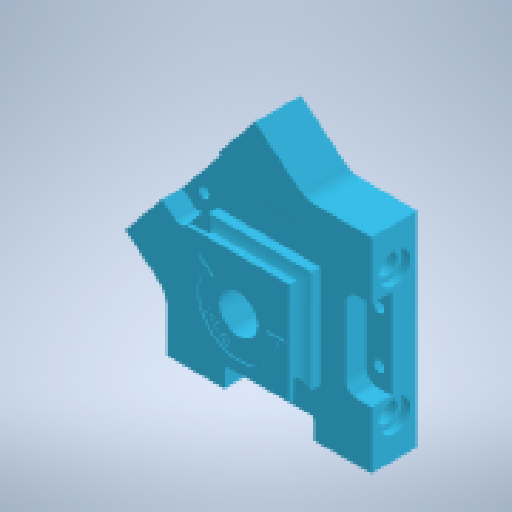
# Autodesk Inventor part: Rail-Angle140.66
Saved by Autodesk Inventor 2023.1 (Build 271208000, 208)
## iProperties
Created: 2023-06-07
Part Number: Rail-Angle140.66
Material: ABS Plastic
Document SubType Name: Modeling
Designer: hello
Density: 1.06 g/cm^3
Appearance: Turquoise
Author: hello
Autodesk Inventor part; units mm, degrees
ref_plane "YZ Plane" through (0, 0, 0) normal (1, 0, 0) x (0, 1, 0)
ref_plane "XZ Plane" through (0, 0, 0) normal (0, 1, 0) x (-1, 0, 0)
ref_plane "XY Plane" through (0, 0, 0) normal (0, 0, 1) x (1, 0, 0)
sketch "Sketch1" plane through (0, 0, 0) normal (0, 0, 1) x (1, 0, 0)
  line L0 (-40, 40) -> (40, 40)
  line L1 (40, 40) -> (40, -40)
  line L2 (40, -40) -> (-40, -40)
  line L3 (-40, -40) -> (-40, 40)
  line L4 (-40, 40) -> (40, -40) construction
  line L5 (40, 40) -> (-40, -40) construction
  line L6 (-56.2928, -5.5791) -> (-5.5791, 56.2928)
  line L7 (40, 0) -> (-40, 0) construction
  line L8 (0, 0) -> (-30.9359, 25.3568) construction
  line L9 (-56.2928, -5.5791) -> (-40, -18.9335)
  line L10 (-5.5791, 56.2928) -> (14.2984, 40)
  dimension "d0" = 80
  dimension "d1" = 80
  dimension "d2" = 80
  dimension "d3" = 140.66
  dimension "d4" = 40
  constraints: 22 end point, 5 midpoint, 4 perpendicular, 2 horizontal, 2 parallel, 2 point on line
  measures "d0" distance of L1.end L2.end
  measures "d1" distance of L0.end L1.end
  measures "d2" distance of L6.start L6.end
  measures "d3" angle of L8 L7
  measures "d4" distance of L8.start L8.end
extrude "Extrusion1" add sketch "Sketch1" along normal blind 18 contours L0 L1 L2 L3 L6 | L0 L6 L10 | L3 L9 L6
sketch "Sketch2" plane through (40, -40, 0) normal (1, 0, 0) x (0, 0, -1)
  line L0 (0, 0) -> (0, 80) projected
  line L1 (0, 80) -> (-18, 80) projected
  line L2 (-18, 0) -> (-18, 80) projected
  line L3 (0, 0) -> (-18, 0) projected
  line L4 (-9, 15) -> (-9, 65)
  point P0 (0, 40)
  point P1 (-9, 40)
  point P2 (0, 40)
  point P3 (-9, 0)
  dimension "d7" = 50
  constraints: 3 midpoint, 2 coincident, 2 end point, 1 horizontal alignment, 1 vertical, 1 vertical alignment
  measures "d7" distance of L4.start L4.end
hole "Hole1" at (40, -25, 9) at (40, 25, 9) direction (-1, 0, 0) diameter 8.05 depth 15 counterbore diameter 12 counterbore depth 3
sketch "Sketch3" plane through (-40, -40, 0) normal (0, -1, 0) x (1, 0, 0)
  line L0 (0, 0) -> (80, 0) projected
  line L1 (80, 0) -> (80, 18) projected
  line L2 (0, 18) -> (80, 18) projected
  line L3 (0, 0) -> (0, 18) projected
  line L4 (15, 9) -> (65, 9)
  point P0 (40, 0)
  point P1 (40, 9)
  point P2 (0, 9)
  point P3 (40, 0)
  dimension "d15" = 50
  constraints: 3 midpoint, 2 coincident, 2 end point, 1 horizontal, 1 horizontal alignment, 1 vertical alignment
  measures "d15" distance of L4.start L4.end
hole "Hole2" at (-25, -40, 9) at (25, -40, 9) direction (0, 1, 0) diameter 8.05 depth 15 counterbore diameter 12 counterbore depth 3
sketch "Sketch4" plane through (0, 0, 18) normal (0, 0, 1) x (1, 0, 0)
  line L0 (40, -40) -> (40, 40) projected
  line L1 (34, -17.5) -> (40, -17.5)
  line L2 (40, -17.5) -> (40, 17.5)
  line L3 (40, 17.5) -> (34, 17.5)
  line L4 (30, 13.5) -> (30, -13.5)
  arc A0 (30, -13.5) -> (34, -17.5) centre (34, -13.5) ccw
  arc A1 (34, 17.5) -> (30, 13.5) centre (34, 13.5) ccw
  point P0 (0, 0)
  point P1 (30, -17.5)
  point P2 (30, 17.5)
  point P3 (40, 0)
  dimension "d23" = 35
  dimension "d24" = 10
  dimension "d25" = 4
  constraints: 8 end point, 4 point on circle, 4 point on line, 4 tangent, 2 centre point, 2 midpoint, 2 parallel, 1 equal radius, 1 horizontal, 1 perpendicular
  measures "d23" distance of point (30, 17.5) point (30, -17.5)
  measures "d24" distance of point (30, -17.5) L1.end
  measures "d25" radius of A0
extrude "Extrusion2" cut sketch "Sketch4" against normal blind 8
sketch "Sketch5" plane through (0, 0, 10) normal (0, 0, 1) x (1, 0, 0)
  line L0 (35, -10) -> (35, 10)
  line L1 (40, 17.5) -> (40, -17.5) projected
  point P0 (0, 0)
  point P1 (35, 0)
  point P2 (40, 0)
  dimension "d28" = 20
  dimension "d29" = 5
  constraints: 2 coincident, 2 end point, 2 midpoint, 1 horizontal alignment, 1 vertical
  measures "d28" distance of L0.start L0.end
  measures "d29" distance between parallel lines of L1 L0
hole "Hole3" at (35, -10, 10) at (35, 10, 10) direction (0, 0, -1) diameter 4 depth 5
pattern_circular "Circular Pattern1" count 2 over 90 about axis through (0, 0, -10) along (0, 0, -1) of "Extrusion2", "Hole3"
sketch "Sketch6" plane through (0, 0, 18) normal (0, 0, 1) x (1, 0, 0)
  line L0 (-20, 20) -> (20, 20)
  line L1 (20, 20) -> (20, -20)
  line L2 (20, -20) -> (-20, -20)
  line L3 (-20, -20) -> (-20, 20)
  line L4 (-20, 20) -> (20, -20) construction
  line L5 (20, 20) -> (-20, -20) construction
  point P0 (0, 0)
  dimension "d40" = 40
  dimension "d41" = 40
  constraints: 12 end point, 2 midpoint, 2 parallel, 1 horizontal, 1 perpendicular
  measures "d40" distance of L1.end L2.end
  measures "d41" distance of L0.end L1.end
extrude "Extrusion3" add sketch "Sketch6" along normal blind 12
sketch "Sketch7" plane through (-56.2928, -5.5791, 0) normal (-0.7733978, 0.633921, 0) x (0, 0, 1)
  line L0 (0, 80) -> (0, 0) projected
  line L1 (0, 0) -> (18, 0) projected
  line L2 (18, 80) -> (18, 0) projected
  line L3 (0, 80) -> (18, 80) projected
  line L4 (9, 65) -> (9, 15)
  point P0 (0, 40)
  point P1 (9, 40)
  point P2 (0, 40)
  point P3 (9, 80)
  dimension "d44" = 50
  constraints: 3 midpoint, 2 coincident, 2 end point, 1 horizontal alignment, 1 vertical, 1 vertical alignment
  measures "d44" distance of L4.start L4.end
hole "Hole4" at (-15.0879, 44.6918, 9) at (-46.7839, 6.0219, 9) direction (0.7733978, -0.633921, 0) diameter 8.05 depth 15 counterbore diameter 12 counterbore depth 3
sketch "Sketch9" plane through (0, 0, 18) normal (0, 0, 1) x (1, 0, 0)
  line L0 (-14.644, 29.4585) -> (-31.7599, 8.5768)
  line L1 (-37.3891, 8.0189) -> (-42.0295, 11.8224)
  line L2 (-42.0295, 11.8224) -> (-19.8423, 38.8913)
  line L3 (-19.8423, 38.8913) -> (-15.2019, 35.0878)
  line L4 (-12.1083, 32.5521) -> (-42.0295, 11.8224) construction
  line L5 (-34.2956, 5.4832) -> (-19.8423, 38.8913) construction
  line L6 (-5.5791, 56.2928) -> (-56.2928, -5.5791) projected
  arc A0 (-14.644, 29.4585) -> (-15.2019, 35.0878) centre (-17.7376, 31.9942) ccw
  arc A1 (-37.3891, 8.0189) -> (-31.7599, 8.5768) centre (-34.8535, 11.1124) ccw
  point P0 (0, 0)
  point P1 (-27.0689, 22.1872)
  point P2 (-30.9359, 25.3568)
  dimension "d52" = 10
  dimension "d53" = 35
  dimension "d56" = 4
  constraints: 12 end point, 4 midpoint, 4 point on circle, 4 point on line, 4 tangent, 2 centre point, 2 parallel, 1 collinear, 1 equal radius, 1 perpendicular
  measures "d52" distance of L5.start L1.end
  measures "d53" distance of L4.start L5.start
  measures "d56" radius of A0
extrude "Extrusion4" cut sketch "Sketch9" against normal blind 8
sketch "Sketch10" plane through (0, 0, 10) normal (0, 0, 1) x (1, 0, 0)
  line L0 (-14.644, 29.4585) -> (-31.7599, 8.5768) projected
  arc A0 (-14.644, 29.4585) -> (-15.2019, 35.0878) centre (-17.7376, 31.9942) ccw projected
  line L1 (-19.8423, 38.8913) -> (-15.2019, 35.0878) projected
  line L2 (-42.0295, 11.8224) -> (-19.8423, 38.8913) projected
  line L3 (-37.3891, 8.0189) -> (-42.0295, 11.8224) projected
  arc A1 (-37.3891, 8.0189) -> (-31.7599, 8.5768) centre (-34.8535, 11.1124) ccw projected
  line L4 (-14.644, 29.4585) -> (-31.7599, 8.5768) projected
  line L5 (-23.2019, 19.0176) -> (-30.9359, 25.3568)
  line L6 (-42.0295, 11.8224) -> (-19.8423, 38.8913) projected
  line L7 (-20.7297, 29.9212) -> (-33.4081, 14.4533)
  point P0 (0, 0)
  point P1 (-27.0689, 22.1872)
  dimension "d57" = 20
  constraints: 4 end point, 4 midpoint, 2 coincident, 1 perpendicular
  measures "d57" distance of L7.start L7.end
hole "Hole5" at (-33.4081, 14.4533, 10) at (-20.7297, 29.9212, 10) direction (0, 0, -1) diameter 4 depth 5
sketch "Sketch11" plane through (-20, -20, 18) normal (0, -1, 0) x (1, 0, 0)
  line L0 (40, 0) -> (0, 0) projected
  line L1 (40, 0) -> (40, 12) projected
  line L2 (0, 12) -> (40, 12) construction
  line L3 (0, 0) -> (0, 12) construction
  line L4 (0, 12) -> (40, 12) projected
  line L5 (0, 12) -> (0, 10)
  line L6 (0, 0) -> (0, 12) projected
  circle A0 centre (0, 6.7947) radius 3 construction
  arc A1 (4.3, 6.7947) -> (0, 10) centre (-2.036, 2.7817) ccw
  arc A2 (0, 3.5894) -> (4.3, 6.7947) centre (-2.036, 10.8077) ccw
  line L7 (3.5, 7.8415) -> (3.5, 5.7479)
  line L8 (0, 10) -> (0, 3.5894)
  point P0 (20, -18)
  point P1 (0, 11)
  dimension "d65" = 2
  dimension "d66" = 6
  dimension "d67" = 7.5
  dimension "d68" = 7.5
  dimension "d69" = 3.5
  dimension "d70" = 4.3
  constraints: 6 end point, 6 point on circle, 3 centre point, 3 point on line, 2 tangent, 2 vertical, 1 horizontal alignment, 1 midpoint
  measures "d65" distance of L2.start L5.end
  measures "d66" diameter of A0
  measures "d67" radius of A1
  measures "d68" radius of A2
  measures "d69" distance from line of L7 point (0, 11)
  measures "d70" distance from line of A1.start L3
extrude "Extrusion5" cut sketch "Sketch11" against normal through all contours L6 A1 L7 A2
pattern_circular "Circular Pattern2" count 4 over 360 about axis through (0, 0, -10) along (0, 0, 1) of "Extrusion5"
fillet "Fillet1" radius 1.5 4 edges at (0, -20, 28) (-20, 0, 28) (0, 20, 28) (20, 0, 28)
fillet "Fillet2" radius 10 2 edges at (-40, -18.9335, 9) (14.2984, 40, 9)
sketch "Sketch12" plane through (0, 0, 30) normal (0, 0, 1) x (1, 0, 0)
  point P0 (0, 0)
  point P1 (0, 0)
  constraints: 1 coincident
hole "Hole6" at (0, 0, 30) direction (0, 0, -1) diameter 5.5 end through all counterbore diameter 15 counterbore depth 20 clearance for "Hex Head Cap Screw ISO 24017" size "M5" standard "ISO"
sketch "Sketch13" plane through (0, 0, 0) normal (0, 0, -1) x (-1, 0, 0)
  line L0 (7.5, -7.5) -> (-7.5, -7.5)
  line L1 (-7.5, -7.5) -> (-7.5, 7.5)
  line L2 (-7.5, 7.5) -> (7.5, 7.5)
  line L3 (7.5, 7.5) -> (7.5, -7.5)
  line L4 (7.5, -7.5) -> (-7.5, 7.5) construction
  line L5 (-7.5, -7.5) -> (7.5, 7.5) construction
  line L6 (-22.5, -22.5) -> (22.5, -22.5)
  line L7 (22.5, -22.5) -> (22.5, 22.5)
  line L8 (22.5, 22.5) -> (-22.5, 22.5)
  line L9 (-22.5, 22.5) -> (-22.5, -22.5)
  point P0 (0, 0)
  dimension "d85" = 15
  dimension "d86" = 15
  dimension "d87" = 15
  constraints: 20 end point, 4 parallel, 2 midpoint, 2 perpendicular, 1 horizontal, 3 other
  measures "d85" distance of L1.end L2.end
  measures "d86" distance of L0.end L1.end
  measures "d87" distance between parallel lines of L0 L6
extrude "Extrusion6" cut sketch "Sketch13" against normal blind 5.5
chamfer "Chamfer1" distance 5.5 angle 45 8 edges at (0, 22.5, 5.5) (22.5, 0, 5.5) (0, -7.5, 5.5) (-7.5, 0, 5.5) (-22.5, 0, 5.5) (0, -22.5, 5.5) (0, 7.5, 5.5) (7.5, 0, 5.5)
sketch "Sketch14" plane through (0, 0, 30) normal (0, 0, 1) x (1, 0, 0)
  circle A0 centre (0, 0) radius 7.5 projected
  line L0 (-20, -20) -> (20, -20) projected
  line L1 (20, -20) -> (20, 20) projected
  line L2 (20, 20) -> (-20, 20) projected
  line L3 (-20, 20) -> (-20, -20) projected
  line L4 (12.5, 0.5) -> (18.5, 0.5)
  line L5 (18.5, 0.5) -> (18.5, -0.5)
  line L6 (18.5, -0.5) -> (12.5, -0.5)
  line L7 (12.5, -0.5) -> (12.5, 0.5)
  line L8 (12.5, 0.5) -> (18.5, -0.5) construction
  line L9 (18.5, 0.5) -> (12.5, -0.5) construction
  line L10 (12.5, 0.5) -> (12.5, 1)
  line L11 (12.5, 1) -> (10.7679, 0)
  line L12 (10.7679, 0) -> (12.5, -1)
  line L13 (12.5, -1) -> (12.5, -0.5)
  line L14 (-14.6248, 11.3408) -> (-9.9844, 7.5373)
  line L15 (-9.9844, 7.5373) -> (-9.3505, 8.3107)
  line L16 (-9.3505, 8.3107) -> (-13.9909, 12.1142)
  line L17 (-13.9909, 12.1142) -> (-14.6248, 11.3408)
  line L18 (-14.6248, 11.3408) -> (-9.3505, 8.3107) construction
  line L19 (-9.9844, 7.5373) -> (-13.9909, 12.1142) construction
  line L20 (-11.9877, 9.8258) -> (0, 0)
  line L21 (-14.6248, 11.3408) -> (-14.9418, 10.9541)
  line L22 (-14.9418, 10.9541) -> (-15.6474, 12.8255)
  line L23 (-15.6474, 12.8255) -> (-13.6739, 12.5009)
  line L24 (-13.6739, 12.5009) -> (-13.9909, 12.1142)
  circle A1 centre (0, 0) radius 2.75 projected
  arc A2 (-13.1553, 8.1968) -> (15.3704, -2) centre (0, 0) ccw construction
  arc A3 (-13.4736, 8.3952) -> (15.7423, -2.0484) centre (0, 0) ccw
  arc A4 (-12.837, 7.9985) -> (14.9986, -1.9516) centre (0, 0) ccw
  arc A5 (-12.837, 7.9985) -> (-13.4736, 8.3952) centre (-13.1553, 8.1968) ccw
  arc A6 (15.7423, -2.0484) -> (14.9986, -1.9516) centre (15.3704, -2) ccw
  point P0 (15.5, 0)
  point P1 (12.5, 0)
  point P2 (20, 0)
  point P3 (-9.6675, 7.924)
  point P4 (-14.3079, 11.7275)
  dimension "d93" = 6
  dimension "d94" = 1
  dimension "d95" = 1.5
  dimension "d97" = 2
  dimension "d98" = 2
  dimension "d99" = 1
  dimension "d100" = 6
  dimension "d101" = 140.66
  dimension "d102" = 15.5
  dimension "d103" = 15.5
  dimension "d104" = 2
  dimension "d106" = 2
  dimension "d107" = 15.5
  dimension "d108" = 0.75
  dimension "d109" = 2
  dimension "d110" = 2
  constraints: 42 end point, 10 point on circle, 9 equal length, 8 midpoint, 5 centre point, 4 tangent, 3 point on line, 2 horizontal alignment, 2 perpendicular, 1 coincident, 1 horizontal, 1 vertical
  measures "d93" distance of L5.end L6.end
  measures "d94" distance of L4.end L5.end
  measures "d95" distance between parallel lines of L1 L5
  measures "d97" distance of L10.end L11.end
  measures "d98" distance of L12.end L10.end
  measures "d99" distance of L15.end L14.end
  measures "d100" distance of L15.end L16.end
  measures "d101" angle of L14 L6
  measures "d102" distance of point (15.5, 0) L20.end
  measures "d103" distance of L20.start L20.end
  measures "d104" distance of L21.end L23.end
  measures "d106" distance of L22.end L23.end
  measures "d107" radius of A2
  measures "d108" radial gap between concentric circles of A3 A4
  measures "d109" distance from line of A2.start L20
  measures "d110" vertical distance of A2.end point (15.5, 0)
extrude "Extrusion7" cut sketch "Sketch14" against normal blind 0.5 contours L4 L5 L6 L7 | L7 L13 L12 L11 L10 | L17 L16 L15 L14 | L21 L22 L23 L24 L17 | A5 A4 A6 A3
sketch "Sketch15" plane through (0, 0, 30) normal (0, 0, 1) x (1, 0, 0)
  line L0 (12.5, 0.5) -> (18.5, 0.5) projected
  line L1 (18.5, 0.5) -> (18.5, -0.5) projected
  line L2 (18.5, -0.5) -> (12.5, -0.5) projected
  line L3 (12.5, -0.5) -> (12.5, -1) projected
  line L4 (12.5, -1) -> (10.7679, 0) projected
  line L5 (10.7679, 0) -> (12.5, 1) projected
  line L6 (12.5, 1) -> (12.5, 0.5) projected
  arc A0 (15.7423, -2.0484) -> (14.9986, -1.9516) centre (15.3704, -2) ccw projected
  arc A1 (-13.4736, 8.3952) -> (15.7423, -2.0484) centre (0, 0) ccw projected
  arc A2 (-12.837, 7.9985) -> (-13.4736, 8.3952) centre (-13.1553, 8.1968) ccw projected
  arc A3 (-12.837, 7.9985) -> (14.9986, -1.9516) centre (0, 0) ccw projected
  line L7 (-14.9418, 10.9541) -> (-15.6474, 12.8255) projected
  line L8 (-15.6474, 12.8255) -> (-13.6739, 12.5009) projected
  line L9 (-13.6739, 12.5009) -> (-13.9909, 12.1142) projected
  line L10 (-13.9909, 12.1142) -> (-9.3505, 8.3107) projected
  line L11 (-9.3505, 8.3107) -> (-9.9844, 7.5373) projected
  line L12 (-9.9844, 7.5373) -> (-14.6248, 11.3408) projected
  line L13 (-14.6248, 11.3408) -> (-14.9418, 10.9541) projected
  circle A4 centre (0, 0) radius 7.5 projected
  line L14 (-20, -20) -> (20, -20) projected
  line L15 (20, -20) -> (20, 20) projected
  line L16 (20, 20) -> (-20, 20) projected
  line L17 (-20, 20) -> (-20, -20) projected
  line L18 (-5.3033, 5.3033) -> (5.3033, -5.3033) construction
  line L19 (5.3033, -5.3033) -> (-3.9842, -14.5908) construction
  line L20 (-3.9842, -14.5908) -> (-14.5908, -3.9842) construction
  line L21 (-14.5908, -3.9842) -> (-5.3033, 5.3033) construction
  line L22 (0, 0) -> (0, 0)
  circle A5 centre (0, 0) radius 2.75 projected
  line L23 (12.5, -1) -> (10.7679, 0) projected
  line L24 (0, 0) -> (10.7679, 0)
  line L25 (-12.3079, -6.1777) -> (-13.3428, -5.1429)
  line L26 (-13.3428, -5.1429) -> (-13.1262, -4.9263)
  line L27 (-13.1262, -4.9263) -> (-12.7411, -5.3113)
  line L28 (-12.7411, -5.3113) -> (-11.3194, -3.8897)
  line L29 (-11.3194, -3.8897) -> (-11.7045, -3.5046)
  line L30 (-11.7045, -3.5046) -> (-11.5103, -3.3103)
  spline S0 degree 2 poles (-11.5103, -3.3103) (-11.2919, -3.5287) (-10.9619, -3.6112) (-10.7762, -3.453) knots 0 0 0 1 2 2 2
  line L31 (-10.7762, -3.453) -> (-10.5562, -3.6731)
  line L32 (-10.5562, -3.6731) -> (-12.4678, -5.5847)
  line L33 (-12.4678, -5.5847) -> (-12.0913, -5.9611)
  line L34 (-12.0913, -5.9611) -> (-12.3079, -6.1777)
  line L35 (-9.8239, -7.204) -> (-10.0766, -6.9513)
  line L36 (-10.0766, -6.9513) -> (-10.8054, -7.6802)
  line L37 (-10.8054, -7.6802) -> (-11.0788, -7.4069)
  line L38 (-11.0788, -7.4069) -> (-10.3499, -6.678)
  line L39 (-10.3499, -6.678) -> (-11.2868, -5.7411)
  line L40 (-11.2868, -5.7411) -> (-10.9877, -5.442)
  line L41 (-10.9877, -5.442) -> (-8.9454, -5.2976)
  line L42 (-8.9454, -5.2976) -> (-8.6841, -5.5589)
  line L43 (-8.6841, -5.5589) -> (-9.8479, -6.7227)
  line L44 (-9.8479, -6.7227) -> (-9.5952, -6.9754)
  line L45 (-9.5952, -6.9754) -> (-9.8239, -7.204)
  line L46 (-10.1213, -6.4493) -> (-9.2927, -5.6208)
  line L47 (-9.2927, -5.6208) -> (-10.8347, -5.7359)
  line L48 (-10.8347, -5.7359) -> (-10.1213, -6.4493)
  spline S1 degree 2 poles (-7.9449, -8.4194) (-8.5157, -8.9901) (-9.3821, -9.193) (-9.7276, -8.8474) knots 0 0 0 1 2 2 2
  spline S2 degree 2 poles (-9.7276, -8.8474) (-10.0783, -8.4967) (-9.8617, -7.6235) (-9.303, -7.0648) knots 0 0 0 1 2 2 2
  spline S3 degree 2 poles (-9.303, -7.0648) (-8.7288, -6.4906) (-7.8658, -6.2912) (-7.5186, -6.6384) knots 0 0 0 1 2 2 2
  spline S4 degree 2 poles (-7.5186, -6.6384) (-7.1696, -6.9874) (-7.3914, -7.8658) (-7.9449, -8.4194) knots 0 0 0 1 2 2 2
  spline S5 degree 2 poles (-8.9557, -8.7013) (-8.8096, -8.6377) (-8.452, -8.3489) (-8.2337, -8.1306) knots 0 0 0 1 2 2 2
  spline S6 degree 2 poles (-8.2337, -8.1306) (-8.0154, -7.9123) (-7.7283, -7.5564) (-7.663, -7.4051) knots 0 0 0 1 2 2 2
  spline S7 degree 2 poles (-7.663, -7.4051) (-7.5977, -7.2539) (-7.6355, -6.9926) (-7.7541, -6.8739) knots 0 0 0 1 2 2 2
  spline S8 degree 2 poles (-7.7541, -6.8739) (-7.8727, -6.7553) (-8.1375, -6.7141) (-8.2939, -6.7811) knots 0 0 0 1 2 2 2
  spline S9 degree 2 poles (-8.2939, -6.7811) (-8.4452, -6.8464) (-8.8062, -7.1456) (-9.0142, -7.3536) knots 0 0 0 1 2 2 2
  spline S10 degree 2 poles (-9.0142, -7.3536) (-9.2377, -7.577) (-9.5093, -7.9037) (-9.5815, -8.0653) knots 0 0 0 1 2 2 2
  spline S11 degree 2 poles (-9.5815, -8.0653) (-9.6502, -8.2165) (-9.6158, -8.4881) (-9.4921, -8.6119) knots 0 0 0 1 2 2 2
  spline S12 degree 2 poles (-9.4921, -8.6119) (-9.3752, -8.7288) (-9.1104, -8.7701) (-8.9557, -8.7013) knots 0 0 0 1 2 2 2
  line L49 (-8.2784, -10.2072) -> (-8.6188, -9.8668)
  line L50 (-8.6188, -9.8668) -> (-8.2131, -9.4611)
  line L51 (-8.2131, -9.4611) -> (-7.8727, -9.8015)
  line L52 (-7.8727, -9.8015) -> (-8.2784, -10.2072)
  spline S13 degree 2 poles (-5.8219, -11.2885) (-5.9852, -11.4518) (-6.3703, -11.6203) (-6.5542, -11.622) knots 0 0 0 1 2 2 2
  spline S14 degree 2 poles (-6.5542, -11.622) (-6.7467, -11.6254) (-7.0854, -11.4896) (-7.2281, -11.3469) knots 0 0 0 1 2 2 2
  spline S15 degree 2 poles (-7.2281, -11.3469) (-7.3708, -11.2043) (-7.51, -10.8725) (-7.5031, -10.6868) knots 0 0 0 1 2 2 2
  spline S16 degree 2 poles (-7.5031, -10.6868) (-7.498, -10.4616) (-7.235, -9.9511) (-6.953, -9.6691) knots 0 0 0 1 2 2 2
  spline S17 degree 2 poles (-6.953, -9.6691) (-6.6763, -9.3924) (-6.1176, -9.0606) (-5.8339, -9.0142) knots 0 0 0 1 2 2 2
  spline S18 degree 2 poles (-5.8339, -9.0142) (-5.5571, -8.9678) (-5.0122, -9.1517) (-4.7733, -9.3907) knots 0 0 0 1 2 2 2
  spline S19 degree 2 poles (-4.7733, -9.3907) (-4.7028, -9.4611) (-4.5928, -9.5987) (-4.5618, -9.6605) knots 0 0 0 1 2 2 2
  line L53 (-4.5618, -9.6605) -> (-4.8351, -9.9339)
  line L54 (-4.8351, -9.9339) -> (-4.8472, -9.9218)
  spline S20 degree 2 poles (-4.8472, -9.9218) (-4.8661, -9.8617) (-4.9744, -9.6812) (-5.0569, -9.5987) knots 0 0 0 1 2 2 2
  spline S21 degree 2 poles (-5.0569, -9.5987) (-5.3216, -9.3339) (-6.0041, -9.3666) (-6.3857, -9.6863) knots 0 0 0 1 2 2 2
  spline S22 degree 2 poles (-6.3857, -9.6863) (-6.2138, -9.7173) (-5.9233, -9.8531) (-5.7961, -9.9803) knots 0 0 0 1 2 2 2
  spline S23 degree 2 poles (-5.7961, -9.9803) (-5.6723, -10.1041) (-5.5365, -10.3396) (-5.5107, -10.5166) knots 0 0 0 1 2 2 2
  spline S24 degree 2 poles (-5.5107, -10.5166) (-5.4815, -10.7212) (-5.6397, -11.1063) (-5.8219, -11.2885) knots 0 0 0 1 2 2 2
  spline S25 degree 2 poles (-6.1227, -11.0117) (-5.9921, -10.8811) (-5.8838, -10.6353) (-5.8975, -10.4977) knots 0 0 0 1 2 2 2
  spline S26 degree 2 poles (-5.8975, -10.4977) (-5.9096, -10.3963) (-6.0213, -10.2261) (-6.0952, -10.1522) knots 0 0 0 1 2 2 2
  spline S27 degree 2 poles (-6.0952, -10.1522) (-6.1949, -10.0525) (-6.4425, -9.9253) (-6.5903, -9.8909) knots 0 0 0 1 2 2 2
  spline S28 degree 2 poles (-6.5903, -9.8909) (-6.623, -9.9201) (-6.6849, -9.9751) (-6.7295, -10.0198) knots 0 0 0 1 2 2 2
  spline S29 degree 2 poles (-6.7295, -10.0198) (-6.9496, -10.2399) (-7.1335, -10.5957) (-7.1387, -10.7315) knots 0 0 0 1 2 2 2
  spline S30 degree 2 poles (-7.1387, -10.7315) (-7.1456, -10.8587) (-7.0682, -11.0427) (-6.9943, -11.1166) knots 0 0 0 1 2 2 2
  spline S31 degree 2 poles (-6.9943, -11.1166) (-6.8224, -11.2885) (-6.3668, -11.2558) (-6.1227, -11.0117) knots 0 0 0 1 2 2 2
  spline S32 degree 2 poles (-4.23, -12.8803) (-4.3933, -13.0437) (-4.7784, -13.2121) (-4.9624, -13.2138) knots 0 0 0 1 2 2 2
  spline S33 degree 2 poles (-4.9624, -13.2138) (-5.1549, -13.2173) (-5.4935, -13.0815) (-5.6362, -12.9388) knots 0 0 0 1 2 2 2
  spline S34 degree 2 poles (-5.6362, -12.9388) (-5.7789, -12.7961) (-5.9182, -12.4643) (-5.9113, -12.2787) knots 0 0 0 1 2 2 2
  spline S35 degree 2 poles (-5.9113, -12.2787) (-5.9061, -12.0535) (-5.6431, -11.5429) (-5.3612, -11.261) knots 0 0 0 1 2 2 2
  spline S36 degree 2 poles (-5.3612, -11.261) (-5.0844, -10.9842) (-4.5257, -10.6524) (-4.2421, -10.606) knots 0 0 0 1 2 2 2
  spline S37 degree 2 poles (-4.2421, -10.606) (-3.9653, -10.5596) (-3.4204, -10.7436) (-3.1814, -10.9825) knots 0 0 0 1 2 2 2
  spline S38 degree 2 poles (-3.1814, -10.9825) (-3.1109, -11.053) (-3.0009, -11.1905) (-2.97, -11.2524) knots 0 0 0 1 2 2 2
  line L55 (-2.97, -11.2524) -> (-3.2433, -11.5257)
  line L56 (-3.2433, -11.5257) -> (-3.2553, -11.5137)
  spline S39 degree 2 poles (-3.2553, -11.5137) (-3.2742, -11.4535) (-3.3825, -11.273) (-3.4651, -11.1905) knots 0 0 0 1 2 2 2
  spline S40 degree 2 poles (-3.4651, -11.1905) (-3.7298, -10.9258) (-4.4123, -10.9584) (-4.7939, -11.2782) knots 0 0 0 1 2 2 2
  spline S41 degree 2 poles (-4.7939, -11.2782) (-4.622, -11.3091) (-4.3315, -11.4449) (-4.2042, -11.5721) knots 0 0 0 1 2 2 2
  spline S42 degree 2 poles (-4.2042, -11.5721) (-4.0805, -11.6959) (-3.9447, -11.9314) (-3.9189, -12.1085) knots 0 0 0 1 2 2 2
  spline S43 degree 2 poles (-3.9189, -12.1085) (-3.8897, -12.3131) (-4.0478, -12.6981) (-4.23, -12.8803) knots 0 0 0 1 2 2 2
  spline S44 degree 2 poles (-4.5309, -12.6036) (-4.4002, -12.4729) (-4.2919, -12.2271) (-4.3057, -12.0896) knots 0 0 0 1 2 2 2
  spline S45 degree 2 poles (-4.3057, -12.0896) (-4.3177, -11.9882) (-4.4294, -11.818) (-4.5034, -11.744) knots 0 0 0 1 2 2 2
  spline S46 degree 2 poles (-4.5034, -11.744) (-4.6031, -11.6443) (-4.8506, -11.5171) (-4.9985, -11.4827) knots 0 0 0 1 2 2 2
  spline S47 degree 2 poles (-4.9985, -11.4827) (-5.0311, -11.512) (-5.093, -11.567) (-5.1377, -11.6117) knots 0 0 0 1 2 2 2
  spline S48 degree 2 poles (-5.1377, -11.6117) (-5.3577, -11.8317) (-5.5417, -12.1876) (-5.5468, -12.3234) knots 0 0 0 1 2 2 2
  spline S49 degree 2 poles (-5.5468, -12.3234) (-5.5537, -12.4506) (-5.4764, -12.6345) (-5.4024, -12.7084) knots 0 0 0 1 2 2 2
  spline S50 degree 2 poles (-5.4024, -12.7084) (-5.2305, -12.8803) (-4.775, -12.8477) (-4.5309, -12.6036) knots 0 0 0 1 2 2 2
  dimension "d113" = 135
  dimension "d114" = 15
  constraints: 4 end point, 2 point on circle, 1 horizontal, 1 midpoint, 2 other
  measures "d113" angle of L24 L22
  measures "d114" distance of L18.start L18.end
emboss "Emboss1" sketch "Sketch15" operation cut depth 0.5 direction (0, 0, -1) contours L25 L26 L27 L28 L29 L30 S0 L31 L32 L33 L34 | L35 L36 L37 L38 L39 L40 L41 L42 L43 L44 L45 | S1 S2 S3 S4 | L49 L50 L51 L52 | S13 S14 S15 S16 S17 S18 S19 L53 L54 S20 S21 S22 S23 S24 | S32 S33 S34 S35 S36 S37 S38 L55 L56 S39 S40 S41 S42 S43
equation "\"d98\" = d97"
equation "\"d103\" = d102"
equation "\"d106\" = d104"
equation "\"d107\" = d102"
body "Solid1"
